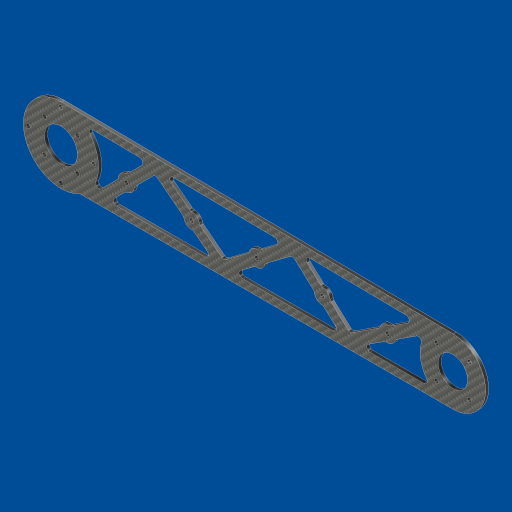
# Autodesk Inventor part: LowerArmPlate
Saved by Autodesk Inventor 2023 (Build 270158030, 158C)
## iProperties
Created: 2023-03-01
Part Number: LowerArmPlate
Material: CFRP
Document SubType Name: Modeling
Designer: kumpu
Density: 1.43 g/cm^3
Appearance: Glossy - Black
Author: kumpu
Autodesk Inventor part; units mm, degrees
ref_plane "YZ Plane" through (0, 0, 0) normal (1, 0, 0) x (0, 1, 0)
ref_plane "XZ Plane" through (0, 0, 0) normal (0, 1, 0) x (-1, 0, 0)
ref_plane "XY Plane" through (0, 0, 0) normal (0, 0, 1) x (1, 0, 0)
sketch "Sketch1" plane through (0, 0, 0) normal (0, 0, 1) x (1, 0, 0)
  line L0 (0, 0) -> (381, 0) construction
  line L1 (0.4564, -36.5096) -> (381.3969, -31.7475)
  line L2 (381.3969, 31.7475) -> (0.4564, 36.5096)
  arc A0 (0.4564, 36.5096) -> (0.4564, -36.5096) centre (0, 0) ccw
  arc A1 (381.3969, -31.7475) -> (381.3969, 31.7475) centre (381, 0) ccw
  circle A2 centre (0, 0) radius 16
  circle A3 centre (381, 0) radius 14.2875
  point P0 (190.5, 0)
  dimension "d0" = 381
  dimension "d2" = 32
  dimension "d5" = 36.5125
  dimension "d6" = 31.75
  dimension "d7" = 28.575
  constraints: 8 end point, 4 centre point, 4 point on circle, 4 tangent, 2 coincident, 1 horizontal, 1 midpoint
  measures "d0" distance of L0.start L0.end
  measures "d2" diameter of A2
  measures "d5" radius of A0
  measures "d6" radius of A1
  measures "d7" diameter of A3
extrude "Extrusion1" add sketch "Sketch1" along normal mid plane 3
sketch "Sketch2" plane through (0, 0, -1.5) normal (0, 0, -1) x (-1, 0, 0)
  circle A0 centre (0, -32) radius 2
  circle A1 centre (-16, -16) radius 2
  line L0 (0, -32) -> (0, 0) construction
  line L1 (0, 0) -> (-16, -16) construction
  line L2 (0, 0) -> (-63.5, 0) construction
  circle A2 centre (-63.5, 0) radius 2
  circle A3 centre (32, 0) radius 2
  circle A4 centre (16, -16) radius 2
  circle A5 centre (0, 32) radius 2
  circle A6 centre (16, 16) radius 2
  circle A7 centre (-32, 0) radius 2
  circle A8 centre (-16, 16) radius 2
  circle A9 centre (-127, 0) radius 2
  circle A10 centre (-190.5, 0) radius 2
  circle A11 centre (-254, 0) radius 2
  circle A12 centre (-317.5, 0) radius 2
  line L3 (-22.684, 28.6112) -> (-84.1585, 27.8427)
  line L4 (-84.1585, 27.8427) -> (-63.924, 7.6082)
  line L5 (-71.1082, 0.424) -> (-91.6778, 20.9935)
  line L6 (-91.6778, 20.9935) -> (-119.3984, -0.5294)
  line L7 (-355.1593, 24.4549) -> (-91.254, 27.754) construction
  line L8 (-0.4564, 36.5096) -> (-381.3969, 31.7475) construction
  line L9 (-39.37, -24.13) -> (-91.254, 27.754) construction
  line L10 (-91.254, 27.754) -> (-158.0785, -24.13) construction
  line L11 (-158.0785, -24.13) -> (-225.5354, 26.0753) construction
  line L12 (-225.5354, 26.0753) -> (-280.341, -24.13) construction
  line L13 (-280.341, -24.13) -> (-355.1593, 24.4549) construction
  line L14 (-39.37, -24.13) -> (-280.341, -24.13) construction
  line L15 (-381.3969, -31.7475) -> (-0.4564, -36.5096) construction
  circle A13 centre (-397, -16) radius 2
  line L16 (-397, -16) -> (-381, 0) construction
  circle A14 centre (-381, 0) radius 14.2875 construction
  circle A15 centre (-365, -16) radius 2
  circle A16 centre (-365, 16) radius 2
  circle A17 centre (-397, 16) radius 2
  line L17 (-315.5033, -7.3537) -> (-289.6687, -24.13)
  line L18 (-289.6687, -24.13) -> (-360.3649, -24.13)
  arc A18 (-360.3649, -24.13) -> (-350.4687, 8.7123) centre (-381, 0) ccw
  arc A19 (-325.0301, -1.1673) -> (-315.5033, -7.3537) centre (-317.5, 0) ccw
  arc A20 (-309.9699, 1.1673) -> (-319.4967, 7.3537) centre (-317.5, 0) ccw
  arc A21 (-253.2434, 7.5823) -> (-261.6195, -0.0906) centre (-254, 0) ccw
  arc A22 (-254.7566, -7.5823) -> (-246.3805, 0.0906) centre (-254, 0) ccw
  arc A23 (-198.0892, -0.6842) -> (-188.9768, -7.4662) centre (-190.5, 0) ccw
  arc A24 (-182.9108, 0.6842) -> (-192.0232, 7.4662) centre (-190.5, 0) ccw
  arc A25 (-125.6293, 7.4957) -> (-134.6016, 0.5294) centre (-127, 0) ccw
  arc A26 (-128.3707, -7.4957) -> (-119.3984, -0.5294) centre (-127, 0) ccw
  arc A27 (-71.1082, 0.424) -> (-63.076, -7.6082) centre (-63.5, 0) ccw
  arc A28 (-55.8918, -0.424) -> (-63.924, 7.6082) centre (-63.5, 0) ccw
  circle A29 centre (-63.5, 0) radius 5.08 construction
  circle A30 centre (-127, 0) radius 5.08 construction
  circle A31 centre (-190.5, 0) radius 5.08 construction
  circle A32 centre (-254, 0) radius 5.08 construction
  circle A33 centre (-317.5, 0) radius 5.08 construction
  line L19 (-319.4967, 7.3537) -> (-346.0079, 24.5693)
  line L20 (-346.0079, 24.5693) -> (-233.16, 25.98)
  line L21 (-233.16, 25.98) -> (-253.2434, 7.5823)
  line L22 (-261.6195, -0.0906) -> (-280.8726, -17.7277)
  line L23 (-280.8726, -17.7277) -> (-309.9699, 1.1673)
  line L24 (-188.9768, -7.4662) -> (-166.587, -24.13)
  line L25 (-166.587, -24.13) -> (-272.8205, -24.13)
  line L26 (-272.8205, -24.13) -> (-254.7566, -7.5823)
  line L27 (-198.0892, -0.6842) -> (-225.2, 19.4932)
  line L28 (-225.2, 19.4932) -> (-246.3805, 0.0906)
  line L29 (-182.9108, 0.6842) -> (-158.1435, -17.7491)
  line L30 (-158.1435, -17.7491) -> (-134.6016, 0.5294)
  line L31 (-125.6293, 7.4957) -> (-99.673, 27.6487)
  line L32 (-99.673, 27.6487) -> (-217.1674, 26.18)
  line L33 (-217.1674, 26.18) -> (-192.0232, 7.4662)
  line L34 (-63.076, -7.6082) -> (-46.5542, -24.13)
  line L35 (-46.5542, -24.13) -> (-149.795, -24.13)
  line L36 (-149.795, -24.13) -> (-128.3707, -7.4957)
  line L37 (-38.9317, -17.3841) -> (-55.8918, -0.424)
  arc A34 (-0.4564, -36.5096) -> (-0.4564, 36.5096) centre (0, 0) ccw construction
  arc A35 (-381.3969, 31.7475) -> (-381.3969, -31.7475) centre (-381, 0) ccw construction
  line L38 (-325.0301, -1.1673) -> (-345.6865, 12.2464)
  arc A36 (-22.684, 28.6112) -> (-33.7517, -13.9279) centre (0, 0) ccw
  arc A37 (-38.9317, -17.3841) -> (-33.7517, -13.9279) centre (-36.6866, -15.1391) ccw
  arc A38 (-345.6865, 12.2464) -> (-350.4687, 8.7123) centre (-347.4156, 9.5836) ccw
  circle A39 centre (-381, 0) radius 24.13 construction
  line L39 (-0.4564, -36.5096) -> (-381.3969, -31.7475)
  arc A40 (-381.3969, -31.7475) -> (-381, -31.75) centre (-381, 0) ccw
  line L40 (-381, -31.75) -> (-18.0305, -31.75)
  arc A41 (-18.0305, -31.75) -> (-0.4564, -36.5096) centre (0, 0) ccw
  dimension "d8" = 45
  dimension "d9" = 16
  dimension "d10" = 32
  dimension "d11" = 4
  dimension "d14" = 360
  dimension "d16" = 63.5
  dimension "d17" = 4
  dimension "d20" = 63.5
  dimension "d26" = 7.62
  dimension "d27" = 45
  dimension "d28" = 45
  dimension "d29" = 16
  dimension "d32" = 360
  dimension "d34" = 10.16
  dimension "d35" = 7.62
  dimension "d36" = 3.175
  constraints: 78 end point, 39 centre point, 32 point on circle, 22 collinear, 21 parallel, 19 equal radius, 19 tangent, 15 concentric, 10 coincident, 8 point on line, 3 horizontal, 1 vertical, 34 other
  measures "d8" angle of L0 L1
  measures "d9" distance from line of L2 L1.end
  measures "d10" distance of L0.start L0.end
  measures "d11" diameter of A0
  measures "d16" distance of L2.end L0.end
  measures "d17" diameter of A2
  measures "d20" distance of A2.centre A9.centre
  measures "d26" distance between parallel lines of L8 L7
  measures "d27" angle of L2 L9
  measures "d28" angle of L2 L16
  measures "d29" horizontal distance of L16.end L16.start
  measures "d34" diameter of A33
  measures "d35" radius of A22
  measures "d36" radius of A37
extrude "Extrusion2" cut sketch "Sketch2" against normal through all
fillet "Fillet1" radius 3.175 37 edges at (22.684, 28.6112, 0) (46.5542, -24.13, 0) (84.1585, 27.8427, 0) (91.6778, 20.9935, 0) (99.673, 27.6487, 0) (55.8918, -0.424, 0) (63.924, 7.6082, 0) (71.1082, 0.424, 0) (63.076, -7.6082, 0) (128.3707, -7.4957, 0) (119.3984, -0.5294, 0) (125.6293, 7.4957, 0) (134.6016, 0.5294, 0) (149.795, -24.13, 0) (158.1435, -17.7491, 0) (166.587, -24.13, 0) (182.9108, 0.6842, 0) (188.9768, -7.4662, 0) (198.0892, -0.6842, 0) (192.0232, 7.4662, 0) (217.1674, 26.18, 0) (225.2, 19.4932, 0) (233.16, 25.98, 0) (246.3805, 0.0906, 0) (253.2434, 7.5823, 0) (261.6195, -0.0906, 0) (254.7566, -7.5823, 0) (272.8205, -24.13, 0) (280.8726, -17.7277, 0) (289.6687, -24.13, 0) (309.9699, 1.1673, 0) (319.4967, 7.3537, 0) (325.0301, -1.1673, 0) (315.5033, -7.3537, 0) (346.0079, 24.5693, 0) (360.3649, -24.13, 0) (18.0305, -31.75, 0)
equation "\"d20\" = d16"
equation "\"d26\" = d25"
equation "\"d25\" = 7.62"
body "Solid1"
